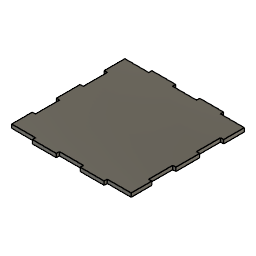
sides-2 (Autodesk Fusion 360 design; units mm, degrees)
part number: 2026-06-16-23-50-00-138
Autodesk Fusion 360 part; units mm, degrees
note: some values were not read from the file. Set by a fixed rule: which sketch regions a step uses.
sketch "Sketch1" plane through (0, 0, 0) normal (0, 0, 1) x (1, 0, 0)
  line L0 (39, 192) -> (77, 192)
  line L1 (77, 192) -> (77, 186)
  line L2 (39, 186) -> (39, 192)
  line L3 (115, 192) -> (153, 192)
  line L4 (153, 192) -> (153, 186)
  line L5 (115, 186) -> (115, 192)
  line L6 (39, 186) -> (0, 186)
  line L7 (77, 186) -> (115, 186)
  line L8 (153, 186) -> (192, 186)
  line L9 (39, 6) -> (0, 6)
  line L10 (39, 6) -> (39, 0)
  line L11 (39, 0) -> (77, 0)
  line L12 (77, 0) -> (77, 6)
  line L13 (77, 6) -> (115, 6)
  line L14 (115, 6) -> (115, 0)
  line L15 (115, 0) -> (153, 0)
  line L16 (153, 0) -> (153, 6)
  line L17 (153, 192) -> (115, 192)
  line L18 (77, 192) -> (39, 192)
  line L19 (39, 0) -> (77, 0)
  line L20 (115, 0) -> (153, 0)
  line L21 (6, 153) -> (0, 153)
  line L22 (0, 153) -> (0, 186)
  line L23 (6, 39) -> (0, 39)
  line L24 (0, 39) -> (0, 6)
  line L25 (0, 115) -> (6, 115)
  line L26 (6, 77) -> (0, 77)
  line L27 (0, 77) -> (0, 115)
  line L28 (6, 39) -> (6, 77)
  line L29 (6, 115) -> (6, 153)
  line L30 (192, 153) -> (192, 186)
  line L31 (186, 153) -> (192, 153)
  line L32 (186, 115) -> (186, 153)
  line L33 (192, 115) -> (186, 115)
  line L34 (192, 77) -> (192, 115)
  line L35 (186, 77) -> (192, 77)
  line L36 (186, 39) -> (186, 77)
  line L37 (186, 39) -> (192, 39)
  line L38 (192, 39) -> (192, 6)
  line L39 (192, 153) -> (192, 186)
  line L40 (192, 6) -> (192, 39)
  line L41 (192, 77) -> (192, 115)
  line L42 (0, 39) -> (0, 6)
  line L43 (0, 186) -> (0, 153)
  line L44 (0, 115) -> (0, 77)
  line L45 (153, 6) -> (192, 6)
  line L46 (5.915, 152.915) -> (-0.085, 152.915)
  line L47 (-0.085, 186.085) -> (-0.085, 152.915)
  line L48 (38.915, 186.085) -> (-0.085, 186.085)
  line L49 (38.915, 186.085) -> (38.915, 192.085)
  line L50 (77.085, 192.085) -> (38.915, 192.085)
  line L51 (77.085, 192.085) -> (77.085, 186.085)
  line L52 (77.085, 186.085) -> (114.915, 186.085)
  line L53 (114.915, 186.085) -> (114.915, 192.085)
  line L54 (114.915, 192.085) -> (153.085, 192.085)
  line L55 (153.085, 192.085) -> (153.085, 186.085)
  line L56 (153.085, 186.085) -> (192.085, 186.085)
  line L57 (192.085, 152.915) -> (192.085, 186.085)
  line L58 (186.085, 152.915) -> (192.085, 152.915)
  line L59 (186.085, 115.085) -> (186.085, 152.915)
  line L60 (192.085, 115.085) -> (186.085, 115.085)
  line L61 (192.085, 76.915) -> (192.085, 115.085)
  line L62 (186.085, 76.915) -> (192.085, 76.915)
  line L63 (186.085, 39.085) -> (186.085, 76.915)
  line L64 (186.085, 39.085) -> (192.085, 39.085)
  line L65 (192.085, 39.085) -> (192.085, 5.915)
  line L66 (153.085, 5.915) -> (192.085, 5.915)
  line L67 (153.085, -0.085) -> (153.085, 5.915)
  line L68 (114.915, -0.085) -> (153.085, -0.085)
  line L69 (114.915, 5.915) -> (114.915, -0.085)
  line L70 (77.085, 5.915) -> (114.915, 5.915)
  line L71 (77.085, -0.085) -> (77.085, 5.915)
  line L72 (38.915, -0.085) -> (77.085, -0.085)
  line L73 (38.915, 5.915) -> (38.915, -0.085)
  line L74 (38.915, 5.915) -> (-0.085, 5.915)
  line L75 (-0.085, 39.085) -> (-0.085, 5.915)
  line L76 (5.915, 39.085) -> (-0.085, 39.085)
  line L77 (5.915, 39.085) -> (5.915, 76.915)
  line L78 (5.915, 76.915) -> (-0.085, 76.915)
  line L79 (-0.085, 115.085) -> (-0.085, 76.915)
  line L80 (-0.085, 115.085) -> (5.915, 115.085)
  line L81 (5.915, 115.085) -> (5.915, 152.915)
  dimension "d3" = 38
  dimension "d4" = 6
  dimension "d5" = 38
  dimension "d6" = 6
  dimension "d7" = 39
  dimension "d8" = 39
  dimension "d10" = 33
  dimension "d12" = 33
  dimension "d13" = 6
  dimension "d14" = 38
  dimension "d15" = 38
  dimension "d16" = 38
  dimension "d19" = 0.085
  constraint horizontal L19
  constraint vertical L40
  constraint horizontal L17
  constraint vertical L43
  constraint horizontal L0
  constraint vertical L1
  constraint vertical L2
  constraint horizontal L3
  constraint vertical L4
  constraint vertical L5
  constraint perpendicular L6 L43
  constraint perpendicular L8 L39
  constraint collinear L17 L18
  constraint collinear L19 L20
  constraint horizontal L21
  constraint vertical L22
  constraint horizontal L23
  constraint vertical L24
  constraint horizontal L25
  constraint horizontal L26
  constraint vertical L27
  constraint perpendicular L26 L28
  constraint collinear L39 L41
  constraint collinear L40 L41
  constraint collinear L42 L44
  constraint collinear L43 L44
  constraint perpendicular L40 L45
  measures "d3" distance of L0.start L0.end
  measures "d4" distance of L0.start L2.start
  measures "d5" distance of L3.start L3.end
  measures "d6" distance of L3.start L5.start
  measures "d7" distance of L4 L39
  measures "d8" distance of L2 L43
  measures "d10" distance of L6.end L21.end
  measures "d12" distance of L9.end L23.end
  measures "d13" distance of L25.start L25.end
  measures "d14" distance of L25.start L26.end
  measures "d15" distance of L21 L25
  measures "d16" distance of L23 L26
extrude "Extrude1" add sketch "Sketch1" along normal blind 6 contours L0 L1 L2 L3 L4 L5 L6 L7 L8 L9 L10 L11 L12 L13 L14 L15 L16 L17 L18 L19 L20 L21 L22 L23 L24 L25 L26 L27 L28 L29 L30 L31 L32 L33 L34 L35 L36 L37 L38 L39 L40 L41 L42 L43 L44 L45
extrude "Extrude2" cut 2 faces at (51.6667, 192, 4) (127.6667, 192, 4) along direction (0, -1, 0) blind 1
extrude "Extrude3" cut 3 faces at (192, 28, 2) (192, 89.6667, 4) (192, 164, 4) along direction (-1, 0, 0) blind 1
extrude "Extrude4" cut 2 faces at (51.6667, 0, 4) (127.6667, 0, 4) along direction (0, 1, 0) blind 1
extrude "Extrude5" cut 3 faces at (0, 164, 4) (0, 89.6667, 4) (0, 28, 2) along direction (1, 0, 0) blind 1
